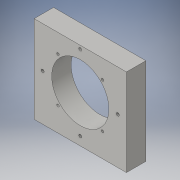
# Autodesk Inventor part: speakerside
Saved by Autodesk Inventor 2016 (Build 200138000, 138)
## iProperties
Created: 2018-09-28
Part Number: speakerside
Material: Generic
Document SubType Name: Modeling
Designer: student
Density: 1 g/cm^3
Appearance: Default
Author: student
Autodesk Inventor part; units mm, degrees
ref_plane "YZ Plane" through (0, 0, 0) normal (1, 0, 0) x (0, 1, 0)
ref_plane "XZ Plane" through (0, 0, 0) normal (0, 1, 0) x (-1, 0, 0)
ref_plane "XY Plane" through (0, 0, 0) normal (0, 0, 1) x (1, 0, 0)
sketch "Sketch1" plane through (0, 0, 0) normal (0, 0, 1) x (1, 0, 0)
  line L0 (0, 0) -> (120.65, 0)
  line L1 (120.65, 0) -> (120.65, 113.919)
  line L2 (0, 113.919) -> (0, 0)
  circle A0 centre (11.2141, 60.325) radius 1.9431
  circle A1 centre (60.325, 11.2141) radius 1.9431
  circle A2 centre (109.4359, 60.325) radius 1.9431
  circle A3 centre (60.325, 109.4359) radius 1.9431
  circle A4 centre (60.325, 60.325) radius 37.3888
  circle A5 centre (31.193, 89.457) radius 1.6129
  circle A6 centre (31.193, 31.193) radius 1.6129
  circle A7 centre (89.457, 31.193) radius 1.6129
  circle A8 centre (89.457, 89.457) radius 1.6129
  line L3 (60.325, 113.919) -> (120.65, 113.919)
  line L4 (60.325, 113.919) -> (0, 113.919)
  dimension "d10" = 3.8862
  dimension "d13" = 360
  dimension "d18" = 74.7776
  dimension "d20" = 3.2258
  dimension "d23" = 360
  dimension "d32" = 4.4831
  constraints: 10 end point, 9 centre point, 2 perpendicular, 1 coincident, 1 horizontal, 1 parallel, 1 point on line, 18 other
  measures "d10" diameter of A0
  measures "d18" diameter of A4
  measures "d20" diameter of A5
  measures "d32" distance from line of L3 A3.centre
extrude "Extrusion3" add sketch "Sketch1" along normal blind 25.4
body "Solid3"
